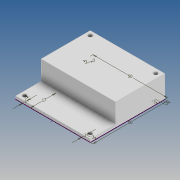
# Autodesk Inventor part: IR pcb shield
Saved by Autodesk Inventor 2020 (Build 240168000, 168)
## iProperties
Created: 2019-08-05
Part Number: IR pcb shield
Material: 일반
Document SubType Name: Modeling
Designer: Chang Ko
Density: 1 g/cm^3
Appearance: 기본값
Author: Chang Ko
## iProperties of the stored document _3D 인쇄.ipt
Created: 2019-08-05
Part Number: _3D 인쇄
Material: 일반
Document SubType Name: Modeling
Designer: Jeong Ji Hoon
Density: 1 g/cm^3
Appearance: 기본값
Author: Jeong Ji Hoon
Autodesk Inventor part; units mm, degrees
ref_plane "YZ Plane" through (0, 0, 0) normal (1, 0, 0) x (0, 1, 0)
ref_plane "XZ Plane" through (0, 0, 0) normal (0, 1, 0) x (-1, 0, 0)
ref_plane "XY Plane" through (0, 0, 0) normal (0, 0, 1) x (1, 0, 0)
sketch "스케치1" plane through (0, 0, 0) normal (0, 1, 0) x (-1, 0, 0)
  line L0 (0, 0) -> (-50, 0)
  line L1 (-50, 0) -> (-50, -17)
  line L2 (-50, -50) -> (0, -50)
  line L3 (0, -50) -> (0, -17)
  line L4 (0, -17) -> (-50, -17)
  line L5 (0, -17) -> (0, 0)
  line L6 (-50, -17) -> (-50, -50)
  point P0 (-25, 0)
  point P1 (-25, -50)
  point P2 (-3, -47)
  point P3 (-47, -47)
  point P4 (-47, -3)
  point P5 (-3, -3)
  dimension "d0" = 50
  dimension "d1" = 50
  dimension "d2" = 17
  dimension "d7" = 3
  dimension "d8" = 3
  dimension "d9" = 3
  dimension "d10" = 3
  dimension "d11" = 3
  dimension "d12" = 3
  dimension "d13" = 3
  dimension "d14" = 3
  constraints: 14 end point, 5 parallel, 4 perpendicular, 2 midpoint, 1 coincident, 1 horizontal
  measures "d0" distance of L2.end L2.start
  measures "d1" distance of L2.start L0.end
  measures "d2" distance between parallel lines of L4 L0
  measures "d7" distance from line of L3 point (-3, -47)
  measures "d8" distance from line of L2 point (-3, -47)
  measures "d9" distance from line of L2 point (-47, -47)
  measures "d10" distance from line of L6 point (-47, -47)
  measures "d11" distance from line of L1 point (-47, -3)
  measures "d12" distance from line of L0 point (-47, -3)
  measures "d13" distance from line of L0 point (-3, -3)
  measures "d14" distance from line of L5 point (-3, -3)
extrude "돌출1" add sketch "스케치1" along normal blind 2 contours L5 L4 L1 L0
extrude "돌출2" add sketch "스케치1" along normal blind 15 contours L3 L2 L6 L4
hole "구멍1" at (3, 0, -47) at (3, 0, -3) at (47, 0, -3) at (47, 0, -47) direction (0, 1, 0) diameter 2.459 end through all thread size "M3x0.5" class "6H" standard "ANSI Metric M Profile"
shell "쉘1" thickness 1 removed faces 1 at (32.0616, 0, -17.9734)
